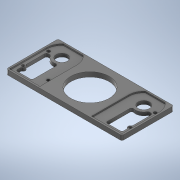
# Autodesk Inventor part: Trunk_upper_waist_frame
Saved by Autodesk Inventor 2020 (Build 240168000, 168)
## iProperties
Created: 2021-09-26
Part Number: Trunk_upper_waist_frame
Material: アセタール樹脂、黒
Document SubType Name: Modeling
Designer: Masato
Density: 1.425 g/cm^3
Appearance: 滑らか - 黒
Mass: 26.3217 g
Surface Area: 125.469 cm^2
Volume: 18.4714 cm^3
Description: POM T5
Author: Masato Kubotera
Autodesk Inventor part; units mm, degrees
ref_plane "YZ Plane" through (0, 0, 0) normal (1, 0, 0) x (0, 1, 0)
ref_plane "XZ Plane" through (0, 0, 0) normal (0, 1, 0) x (-1, 0, 0)
ref_plane "XY Plane" through (0, 0, 0) normal (0, 0, 1) x (1, 0, 0)
derived "Trunk_basis_frame.ipt"
sketch "スケッチ1" plane through (0, 0, 0) normal (0, 0, 1) x (1, 0, 0)
  line L0 (-62, 30.75) -> (62, 30.75) construction
  line L1 (62, -30.75) -> (-62, -30.75) construction
  line L2 (-62, 30.75) -> (62, -30.75) construction
  line L3 (62, 30.75) -> (-62, -30.75) construction
  line L4 (0, 30.75) -> (0, -30.75) construction
  circle A0 centre (-44, 2.25) radius 10.5 construction
  line L5 (-57.5, 1.25) -> (-30.5, 1.25) construction
  line L6 (-30.5, 1.25) -> (-30.5, -25.75) construction
  line L7 (-30.5, -25.75) -> (-57.5, -25.75) construction
  line L8 (-57.5, -25.75) -> (-57.5, 1.25) construction
  line L9 (-44, 1.25) -> (-44, -25.75) construction
  line L10 (-57.5, -12.25) -> (-30.5, -12.25) construction
  circle A1 centre (-57.5, 1.25) radius 1.5 construction
  circle A2 centre (-57.5, -25.75) radius 1.5
  circle A3 centre (-30.5, 1.25) radius 1.5 construction
  circle A4 centre (-30.5, -25.75) radius 1.5
  line L11 (-27.5, 14.75) -> (-22.5, 14.75) construction
  line L12 (-22.5, 14.75) -> (-22.5, -10.25) construction
  line L13 (-22.5, -10.25) -> (-27.5, -10.25) construction
  line L14 (-27.5, -10.25) -> (-27.5, 14.75) construction
  line L15 (-27.5, 14.75) -> (-22.5, -10.25) construction
  line L16 (-22.5, 14.75) -> (-27.5, -10.25) construction
  line L17 (-27.51, 14.76) -> (-22.49, 14.76) construction
  line L18 (-22.49, 14.76) -> (-22.49, -10.26) construction
  line L19 (-22.49, -10.26) -> (-27.51, -10.26) construction
  line L20 (-27.51, -10.26) -> (-27.51, 14.76) construction
  line L21 (-27.51, 14.76) -> (-22.49, -10.26) construction
  line L22 (-22.49, 14.76) -> (-27.51, -10.26) construction
  line L23 (-27.51, 2.25) -> (-22.49, 2.25) construction
  line L24 (-25, 14.76) -> (-25, -10.26) construction
  arc A5 (-27.51, 14.76) -> (-27.51, 12.66) centre (-27.51, 13.71) ccw construction
  arc A6 (-22.49, 12.66) -> (-22.49, 14.76) centre (-22.49, 13.71) ccw construction
  arc A7 (-22.49, -10.26) -> (-22.49, -8.16) centre (-22.49, -9.21) ccw construction
  arc A8 (-27.51, -8.16) -> (-27.51, -10.26) centre (-27.51, -9.21) ccw construction
  circle A9 centre (-25, 27.75) radius 1.55 construction
  line L25 (-22.5, -17.25) -> (-27.5, -17.25) construction
  circle A10 centre (-25, -23.25) radius 1.55 construction
  circle A11 centre (-44, 2.25) radius 11 construction
  line L26 (62, 2.25) -> (-62, 2.25) construction
  line L27 (-60, 14.25) -> (-28, 14.25) construction
  line L28 (-28, 14.25) -> (-28, -28.75) construction
  line L29 (-28, -28.75) -> (-60, -28.75) construction
  line L30 (-60, -28.75) -> (-60, 14.25) construction
  line L31 (-60, 14.25) -> (-28, -28.75) construction
  line L32 (-28, 14.25) -> (-60, -28.75) construction
  line L33 (-62, 30.75) -> (-62, -30.75) construction
  line L34 (62, 30.75) -> (62, -30.75) construction
  circle A12 centre (-44, 2.25) radius 12.5 construction
  circle A13 centre (-44, 2.25) radius 20.5 construction
  circle A14 centre (-44, 2.25) radius 28.5 construction
  circle A15 centre (-44, 26.75) radius 1.25 construction
  circle A16 centre (-61.3241, 19.5741) radius 1.25 construction
  circle A17 centre (-68.5, 2.25) radius 1.25 construction
  circle A18 centre (-61.3241, -15.0741) radius 1.25 construction
  circle A19 centre (-44, -22.25) radius 1.25 construction
  circle A20 centre (-26.6759, -15.0741) radius 1.25 construction
  circle A21 centre (-19.5, 2.25) radius 1.25 construction
  circle A22 centre (-26.6759, 19.5741) radius 1.25 construction
  line L35 (-62, -21.122) -> (-62, -30.75) construction
  circle A23 centre (26.6759, -15.0741) radius 1.25 construction
  circle A24 centre (25, -23.25) radius 1.55 construction
  circle A25 centre (30.5, -25.75) radius 1.5 construction
  circle A26 centre (44, -22.25) radius 1.25 construction
  circle A27 centre (57.5, -25.75) radius 1.5
  circle A28 centre (61.3241, -15.0741) radius 1.25 construction
  line L36 (62, -21.122) -> (62, -30.75) construction
  circle A29 centre (68.5, 2.25) radius 1.25 construction
  circle A30 centre (61.3241, 19.5741) radius 1.25 construction
  circle A31 centre (44, 26.75) radius 1.25 construction
  circle A32 centre (44, 2.25) radius 11 construction
  circle A33 centre (26.6759, 19.5741) radius 1.25 construction
  circle A34 centre (25, 27.75) radius 1.55 construction
  circle A35 centre (30.5, 1.25) radius 1.5 construction
  circle A36 centre (57.5, 1.25) radius 1.5 construction
  circle A37 centre (19.5, 2.25) radius 1.25 construction
  line L37 (22.49, -10.26) -> (27.51, -10.26) construction
  arc A38 (27.51, -10.26) -> (27.51, -8.16) centre (27.51, -9.21) ccw construction
  arc A39 (22.49, -8.16) -> (22.49, -10.26) centre (22.49, -9.21) ccw construction
  line L38 (22.49, 14.76) -> (22.49, -10.26) construction
  line L39 (27.51, -10.26) -> (27.51, 14.76) construction
  arc A40 (22.49, 14.76) -> (22.49, 12.66) centre (22.49, 13.71) ccw construction
  line L40 (27.51, 14.76) -> (22.49, 14.76) construction
  arc A41 (27.51, 12.66) -> (27.51, 14.76) centre (27.51, 13.71) ccw construction
  line L41 (-68.5, 2.25) -> (-73.5, 2.25) construction
  circle A42 centre (-26.6759, -15.0741) radius 6.25 construction
  circle A43 centre (-44, 2.25) radius 24.5 construction
  circle A44 centre (-30.5, -25.75) radius 2.4 construction
  line L42 (-62, 16.25) -> (62, 16.25)
  line L43 (-60.25, 2.25) -> (-60.25, -36.0151)
  circle A45 centre (-44, 2.25) radius 6.05
  arc A46 (-54.6771, 14.5) -> (-55.2379, 13.9876) centre (-44, 2.25) ccw construction
  line L44 (-54.6771, 14.5) -> (-53.9174, 14.5) construction
  arc A47 (-53.9174, 14.5) -> (-55.2379, 13.9876) centre (-54.2972, 13.5211) ccw
  arc A48 (-55.2379, 13.9876) -> (-60.25, 2.25) centre (-44, 2.25) ccw
  line L45 (-60.25, -37.5) -> (-58.7651, -37.5) construction
  arc A49 (-60.25, -36.0151) -> (-58.7651, -37.5) centre (-59.5075, -36.7575) ccw
  line L46 (-60.25, -36.0151) -> (-60.25, -37.5) construction
  line L47 (-58.7651, -37.5) -> (-29.2349, -37.5)
  arc A50 (-57.5, 2.75) -> (-57.5, -0.25) centre (-57.5, 1.25) ccw
  arc A51 (-57, -0.25) -> (-57, 2.75) centre (-57, 1.25) ccw
  line L48 (-57.5, 2.75) -> (-57, 2.75)
  line L49 (-57.5, -0.25) -> (-57, -0.25)
  line L50 (-27.75, 2.25) -> (-27.75, -36.0151)
  arc A52 (-32.7621, 13.9876) -> (-34.0826, 14.5) centre (-33.7028, 13.5211) ccw
  arc A53 (-27.75, 2.25) -> (-32.7621, 13.9876) centre (-44, 2.25) ccw
  arc A54 (-29.2349, -37.5) -> (-27.75, -36.0151) centre (-28.4925, -36.7575) ccw
  line L51 (-53.9174, 14.5) -> (-34.0826, 14.5)
  arc A55 (-52.3331, -1.15) -> (-39.5, -5.5442) centre (-44, 2.25) ccw
  line L52 (-52.3331, -1.15) -> (-57, -1.15)
  line L53 (-57, -1.15) -> (-57, -23.4027)
  line L54 (60.25, 2.25) -> (60.25, -36.0151)
  circle A56 centre (44, 2.25) radius 6.05
  arc A57 (55.2379, 13.9876) -> (53.9174, 14.5) centre (54.2972, 13.5211) ccw
  arc A58 (60.25, 2.25) -> (55.2379, 13.9876) centre (44, 2.25) ccw
  arc A59 (58.7651, -37.5) -> (60.25, -36.0151) centre (59.5075, -36.7575) ccw
  line L55 (58.7651, -37.5) -> (29.2349, -37.5)
  arc A60 (57.5, -0.25) -> (57.5, 2.75) centre (57.5, 1.25) ccw
  arc A61 (57, 2.75) -> (57, -0.25) centre (57, 1.25) ccw
  line L56 (57.5, 2.75) -> (57, 2.75)
  arc A62 (32.7621, 13.9876) -> (27.75, 2.25) centre (44, 2.25) ccw
  arc A63 (34.0826, 14.5) -> (32.7621, 13.9876) centre (33.7028, 13.5211) ccw
  line L57 (27.75, 2.25) -> (27.75, -36.0151)
  arc A64 (27.75, -36.0151) -> (29.2349, -37.5) centre (28.4925, -36.7575) ccw
  line L58 (53.9174, 14.5) -> (34.0826, 14.5)
  arc A65 (39.5, -5.5442) -> (52.3331, -1.15) centre (44, 2.25) ccw
  line L59 (52.3331, -1.15) -> (57, -1.15)
  line L60 (57, -1.15) -> (57, -23.4027)
  line L61 (57.5, -0.25) -> (57, -0.25)
  circle A66 centre (0, -11.5) radius 20.5
  arc A67 (-57, -28.0973) -> (-57, -23.4027) centre (-57.5, -25.75) ccw
  line L62 (-57, -28.0973) -> (-57, -34.25)
  line L63 (-57, -34.25) -> (-39.5, -34.25)
  line L64 (-39.5, -34.25) -> (-39.5, -5.5442)
  arc A68 (57, -23.4027) -> (57, -28.0973) centre (57.5, -25.75) ccw
  line L65 (57, -28.0973) -> (57, -34.25)
  line L66 (57, -34.25) -> (39.5, -34.25)
  line L67 (39.5, -34.25) -> (39.5, -5.5442)
  line L68 (-62, 16.25) -> (-62, -39.25)
  line L69 (-62, -39.25) -> (62, -39.25)
  line L70 (62, -39.25) -> (62, 16.25)
  line L71 (-60, -37.25) -> (-28, -37.25) construction
  arc A69 (-47.969, 27.2469) -> (-58.8689, 22.732) centre (-44, 2.25) ccw
  arc A70 (-44, 30.75) -> (-47.969, 27.2469) centre (-44, 26.75) ccw
  arc A71 (-58.8689, 22.732) -> (-64.482, 17.1189) centre (-61.3241, 19.5741) ccw
  arc A72 (-64.482, 17.1189) -> (-68.9969, 6.219) centre (-44, 2.25) ccw
  arc A73 (-68.9969, 6.219) -> (-68.9969, -1.719) centre (-68.5, 2.25) ccw
  arc A74 (-68.9969, -1.719) -> (-64.482, -12.6189) centre (-44, 2.25) ccw
  arc A75 (-64.482, -12.6189) -> (-62, -19.0166) centre (-61.3241, -15.0741) ccw
  line L72 (-62, -19.0166) -> (-62, -21.122)
  arc A76 (47.969, 27.2469) -> (44, 30.75) centre (44, 26.75) ccw
  arc A77 (58.8689, 22.732) -> (47.969, 27.2469) centre (44, 2.25) ccw
  arc A78 (64.482, 17.1189) -> (58.8689, 22.732) centre (61.3241, 19.5741) ccw
  arc A79 (68.9969, 6.219) -> (64.482, 17.1189) centre (44, 2.25) ccw
  arc A80 (68.9969, -1.719) -> (68.9969, 6.219) centre (68.5, 2.25) ccw
  arc A81 (64.482, -12.6189) -> (68.9969, -1.719) centre (44, 2.25) ccw
  arc A82 (62, -19.0166) -> (64.482, -12.6189) centre (61.3241, -15.0741) ccw
  line L73 (62, -19.0166) -> (62, -21.122)
  line L74 (19.5, 25.75) -> (-19.5, 25.75)
  line L75 (-19.5, 25.75) -> (-19.5, 7.25)
  circle A83 centre (-25, 27.75) radius 2.75 construction
  line L76 (-15.1699, 4.75) -> (15.1699, 4.75)
  arc A84 (-15.1699, 4.75) -> (-19.5, 7.25) centre (-19.5, 2.25) ccw
  line L77 (19.5, 25.75) -> (19.5, 7.25)
  arc A85 (19.5, 7.25) -> (15.1699, 4.75) centre (19.5, 2.25) ccw
  arc A86 (-19.5, -2.75) -> (-15.1699, -0.25) centre (-19.5, 2.25) ccw
  line L78 (-15.1699, -0.25) -> (15.1699, -0.25)
  arc A87 (15.1699, -0.25) -> (19.5, -2.75) centre (19.5, 2.25) ccw
  line L79 (-19.5, -2.75) -> (-19.5, -25.75)
  line L80 (-19.5, -25.75) -> (19.5, -25.75)
  line L81 (19.5, -25.75) -> (19.5, -2.75)
  point P0 (0, 0)
  point P1 (-25, 2.25)
  point P2 (-44, -7.25)
  point P3 (28, -28.75)
  point P4 (-25, 2.25)
  point P5 (-22.49, 12.66)
  point P6 (-22.49, -8.16)
  point P7 (-27.51, -8.16)
  point P8 (22.49, -8.16)
  point P9 (22.49, 12.66)
  point P10 (27.9147, 19.7411)
  point P11 (27.51, 18.6431)
  point P12 (27.51, -8.16)
  point P13 (-27.51, 18.6431)
  point P14 (-27.9147, 19.7411)
  point P15 (-26.4271, 21.76)
  point P16 (-26.9247, 21.76)
  point P17 (-27.51, 20.5051)
  point P18 (27.51, 20.5051)
  point P19 (26.9247, 21.76)
  point P20 (26.4271, 21.76)
  point P21 (-47, 30.75)
  point P22 (47, 30.75)
  dimension "d6" = 12.1
  dimension "d7" = 0.25
  dimension "d9" = 0.25
  dimension "d10" = 1.05
  dimension "d11" = 1.05
  dimension "d13" = 0.5
  dimension "d14" = 16.25
  dimension "d16" = 9
  dimension "d17" = 2.4
  dimension "d18" = 5
  dimension "d21" = 2
  dimension "d22" = 2
  dimension "d24" = 7.25
  dimension "d27" = 2.4
  dimension "d29" = 8.5
  dimension "d30" = 0.25
  dimension "d31" = 2
  dimension "d32" = 5
  dimension "d35" = 55.5
  dimension "d41" = 12
  dimension "d42" = 41
  measures "d6" diameter of A45
  measures "d7" distance between parallel lines of L43 L30
  measures "d9" distance between parallel lines of L27 L44
  measures "d10" radius of A47
  measures "d11" radius of A49
  measures "d13" distance of A1.centre A51.centre
  measures "d14" radius of A48
  measures "d16" radius of A55
  measures "d17" distance of L52.end A51.centre
  measures "d18" horizontal distance of L1.end L53.end
  measures "d21" horizontal distance of L42.start L27.start
  measures "d22" horizontal distance of L42.start L27.start
  measures "d24" distance edge to line of A66 L42
  measures "d27" radius of A67
  measures "d29" distance of L71.start L29.end
  measures "d30" horizontal distance of L45.start L71.start
  measures "d31" horizontal distance of L68.end L71.start
  measures "d32" horizontal distance of L68.end L62.end
  measures "d35" distance of L68.end L42.start
  measures "d41" distance between parallel lines of L64 L14
  measures "d42" diameter of A66
extrude "押し出し1" add sketch "スケッチ1" along normal blind 5 contours L42 L75 A84 L76 A66 A86 L79 L80 L81 A87 A85 L77 L70 L69 L68 | L42 L77 A85 L76 A66 A84 L75 | A66 L79 A86 | A87 L81 A66 | A66 L80 L79 | L81 L80 A66
extrude "押し出し2" add sketch "スケッチ1" along normal blind 3.5 contours A48 A47 L51 A52 A53 L50 A54 L47 A49 L43 | L54 A59 L55 A64 L57 A62 A63 L58 A57 A58
fillet "フィレット1" radius 2 18 edges at (-62, 16.25, 2.5) (-62, -39.25, 2.5) (-52.3331, -1.15, 1.75) (-57, -1.15, 1.75) (-39.5, -5.5442, 1.75) (-39.5, -34.25, 1.75) (-57, -34.25, 1.75) (39.5, -34.25, 1.75) (39.5, -5.5442, 1.75) (62, -39.25, 2.5) (62, 16.25, 2.5) (52.3331, -1.15, 1.75) (57, -1.15, 1.75) (57, -34.25, 1.75) (-57, -23.4027, 1.75) (-57, -28.0973, 1.75) (57, -23.4027, 1.75) (57, -28.0973, 1.75)
equation "\"d9\" = d7"
equation "\"d21\" = d22"
equation "\"d24\" = -0.5 * d26 + 0.5 * d35"
equation "\"d30\" = d7"
equation "\"d31\" = d22"
equation "\"d32\" = d18"
equation "\"d26\" = 41"
